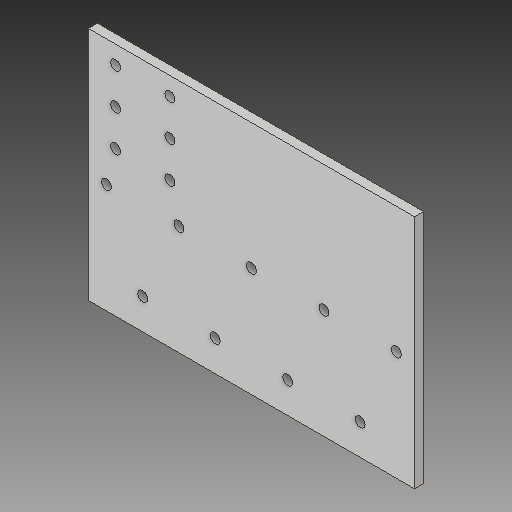
# Autodesk Inventor part: GantryPlate_v3
Saved by Autodesk Inventor 2017 (Build 210142000, 142)
## iProperties
Created: 2017-03-29
Part Number: GantryPlate_v3
Material: Generic
Document SubType Name: Modeling
Designer: Ali
Density: 1 g/cm^3
Appearance: Default
Author: Ali
Autodesk Inventor part; units mm, degrees
ref_plane "YZ Plane" through (0, 0, 0) normal (1, 0, 0) x (0, 1, 0)
ref_plane "XZ Plane" through (0, 0, 0) normal (0, 1, 0) x (-1, 0, 0)
ref_plane "XY Plane" through (0, 0, 0) normal (0, 0, 1) x (1, 0, 0)
sketch "Sketch1" plane through (0, 0, 0) normal (0, 0, 1) x (1, 0, 0)
  line L0 (0, 0) -> (180, 0)
  line L1 (180, 0) -> (180, -130)
  line L2 (180, -130) -> (0, -130)
  line L3 (0, -130) -> (0, 0)
  dimension "d0" = 180
  dimension "d1" = 130
  constraints: 8 end point, 2 parallel, 1 horizontal, 1 perpendicular
  measures "d0" distance of L1.end L2.end
  measures "d1" distance of L0.end L1.end
extrude "Extrusion1" add sketch "Sketch1" along normal blind 5
sketch "Sketch2" plane through (0, 0, 5) normal (0, 0, 1) x (1, 0, 0)
  line L0 (0, -130) -> (180, -130) projected
  line L1 (180, -130) -> (150, -130)
  line L2 (150, -130) -> (150, -113)
  circle A0 centre (150, -113) radius 2.75
  line L3 (180, -130) -> (180, 0) projected
  line L4 (180, -69.5) -> (170, -69.5)
  line L5 (180, -69.5) -> (190, -69.5) construction
  circle A1 centre (170, -69.5) radius 2.75
  circle A2 centre (130, -69.5) radius 2.75
  circle A3 centre (90, -69.5) radius 2.75
  circle A4 centre (50, -69.5) radius 2.75
  circle A5 centre (10, -69.5) radius 2.75
  circle A6 centre (110, -113) radius 2.75
  circle A7 centre (70, -113) radius 2.75
  circle A8 centre (30, -113) radius 2.75
  point P0 (0, 0)
  dimension "d4" = 30
  dimension "d6" = 5.5
  dimension "d25" = 10
  dimension "d26" = 180
  dimension "d33" = 5.5
  dimension "d34" = 5.5
  dimension "d35" = 5.5
  dimension "d37" = 5.5
  dimension "d53" = 43.5
  dimension "d56" = 40
  constraints: 9 centre point, 8 end point, 3 horizontal, 2 coincident, 2 point on line, 1 collinear, 1 perpendicular, 6 other
  measures "d4" distance of L0.end L1.end
  measures "d6" diameter of A0
  measures "d25" distance of L4.start L4.end
  measures "d26" angle of L4 L5
  measures "d33" diameter of A1
  measures "d34" diameter of A2
  measures "d35" diameter of A3
  measures "d37" diameter of A5
  measures "d53" vertical distance of L2.end L4.end
  measures "d56" distance of A0.centre A6.centre
extrude "Extrusion2" cut sketch "Sketch2" against normal blind 5
sketch "Sketch3" plane through (0, 0, 5) normal (0, 0, 1) x (1, 0, 0)
  line L0 (0, 0) -> (180, 0) projected
  line L1 (0, 0) -> (15, 0)
  line L2 (15, 0) -> (15, -10)
  circle A0 centre (15, -10) radius 2.75
  line L3 (15, -10) -> (15, -30)
  line L4 (15, -30) -> (15, -50)
  circle A1 centre (15, -30) radius 2.75
  circle A2 centre (15, -50) radius 2.75
  line L5 (15, -10) -> (45, -10)
  line L6 (45, -10) -> (45, -30)
  line L7 (45, -30) -> (45, -50)
  circle A3 centre (45, -10) radius 2.75
  circle A4 centre (45, -30) radius 2.75
  circle A5 centre (45, -50) radius 2.75
  dimension "d40" = 15
  dimension "d41" = 10
  dimension "d42" = 5.5
  dimension "d43" = 20
  dimension "d44" = 20
  dimension "d45" = 5.5
  dimension "d46" = 5.5
  dimension "d47" = 30
  dimension "d48" = 5.5
  dimension "d49" = 5.5
  dimension "d50" = 5.5
  constraints: 14 end point, 6 centre point, 6 coincident, 3 point on line, 2 perpendicular, 1 horizontal, 1 vertical
  measures "d40" distance of L0.start L1.end
  measures "d41" distance of L1.end L2.end
  measures "d42" diameter of A0
  measures "d43" distance of L3.start L3.end
  measures "d44" distance of L3.end L4.end
  measures "d45" diameter of A1
  measures "d46" diameter of A2
  measures "d47" distance of L3.start L5.end
  measures "d48" diameter of A3
  measures "d49" diameter of A4
  measures "d50" diameter of A5
extrude "Extrusion3" cut sketch "Sketch3" against normal blind 5
body "Solid1"
